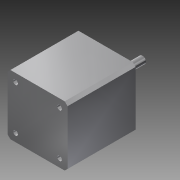
# Autodesk Inventor part: nema17
Saved by Autodesk Inventor 2014 SP2 (Build 180246200, 246)
## iProperties
Created: 2014-07-14
Part Number: nema17
Material: Generic
Document SubType Name: Modeling
Designer: cruiser
Density: 1 g/cm^3
Appearance: Silver
Author: cruiser
Autodesk Inventor part; units mm, degrees
ref_plane "YZ Plane" through (0, 0, 0) normal (1, 0, 0) x (0, 1, 0)
ref_plane "XZ Plane" through (0, 0, 0) normal (0, 1, 0) x (-1, 0, 0)
ref_plane "XY Plane" through (0, 0, 0) normal (0, 0, 1) x (1, 0, 0)
sketch "Sketch1" plane through (0, 0, 0) normal (0, 1, 0) x (-1, 0, 0)
  line L0 (19.15, -21.15) -> (-19.15, -21.15)
  line L1 (-21.15, -19.15) -> (-21.15, 19.15)
  line L2 (-19.15, 21.15) -> (19.15, 21.15)
  line L3 (21.15, 19.15) -> (21.15, -19.15)
  line L4 (21.15, -21.15) -> (-21.15, 21.15) construction
  line L5 (-21.15, -21.15) -> (21.15, 21.15) construction
  line L6 (-19.15, 21.15) -> (-21.15, 19.15)
  line L7 (-19.15, -21.15) -> (-21.15, -19.15)
  line L8 (19.15, -21.15) -> (21.15, -19.15)
  line L9 (19.15, 21.15) -> (21.15, 19.15)
  point P0 (0, 0)
  dimension "d0" = 42.3
  dimension "d1" = 42.3
  dimension "d2" = 2
  dimension "d3" = 2
  dimension "d4" = 2
  dimension "d5" = 2
  dimension "d6" = 2
  dimension "d7" = 2
  dimension "d8" = 2
  dimension "d9" = 2
  constraints: 20 end point, 8 point on line, 2 midpoint, 2 parallel, 1 horizontal, 1 perpendicular
  measures "d0" distance of L4.end L5.end
  measures "d1" distance of L5.start L4.end
  measures "d2" distance of L2.start L4.end
  measures "d3" distance of L1.end L4.end
  measures "d4" distance of L0.end L5.start
  measures "d5" distance of L1.start L5.start
  measures "d6" distance of L0.start L4.start
  measures "d7" distance of L3.end L4.start
  measures "d8" distance of L2.end L5.end
  measures "d9" distance of L3.start L5.end
extrude "Extrusion1" add sketch "Sketch1" along normal blind 48
sketch "Sketch3" plane through (0, 48, 0) normal (0, 1, 0) x (1, 0, 0)
  line L0 (15.5, -15.5) -> (-15.5, -15.5)
  line L1 (-15.5, -15.5) -> (-15.5, 15.5)
  line L2 (-15.5, 15.5) -> (15.5, 15.5)
  line L3 (15.5, 15.5) -> (15.5, -15.5)
  line L4 (15.5, -15.5) -> (-15.5, 15.5) construction
  line L5 (-15.5, -15.5) -> (15.5, 15.5) construction
  circle A0 centre (-15.5, 15.5) radius 1.65
  circle A1 centre (15.5, 15.5) radius 1.65
  circle A2 centre (-15.5, -15.5) radius 1.65
  circle A3 centre (15.5, -15.5) radius 1.65
  point P0 (0, 0)
  dimension "d15" = 31
  dimension "d16" = 31
  dimension "d17" = 3.3
  dimension "d18" = 3.3
  dimension "d19" = 3.3
  dimension "d20" = 3.3
  constraints: 12 end point, 4 centre point, 4 coincident, 2 midpoint, 2 parallel, 1 horizontal, 1 perpendicular
  measures "d15" distance of L1.end L2.end
  measures "d16" distance of L0.end L1.end
  measures "d17" diameter of A0
  measures "d18" diameter of A1
  measures "d19" diameter of A2
  measures "d20" diameter of A3
hole "Hole1" at (15.5, 48, -15.5) at (15.5, 48, 15.5) at (-15.5, 48, 15.5) at (-15.5, 48, -15.5) direction (0, -1, 0) diameter 3.3 end through all
sketch "Sketch2" plane through (0, 48, 0) normal (0, 1, 0) x (1, 0, 0)
  circle A0 centre (0, 0) radius 11
  dimension "d12" = 22
  constraints: 1 centre point, 1 coincident
  measures "d12" diameter of A0
extrude "Extrusion2" add sketch "Sketch2" along normal blind 2
sketch "Sketch4" plane through (0, 50, 0) normal (0, 1, 0) x (1, 0, 0)
  circle A0 centre (0, 0) radius 11 projected
  circle A1 centre (0, 0) radius 2.5
  dimension "d28" = 5
  constraints: 1 centre point, 1 coincident
  measures "d28" diameter of A1
extrude "Extrusion3" add sketch "Sketch4" along normal blind 24 contours A1
equation "\"d3\" = d2"
equation "\"d4\" = d2"
equation "\"d5\" = d4"
equation "\"d6\" = d2"
equation "\"d7\" = d6"
equation "\"d8\" = d2"
equation "\"d9\" = d8"
body "Solid1"
